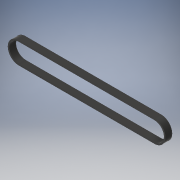
# Autodesk Inventor part: BeltVer1-1111-2019
Saved by Autodesk Inventor 2018 (Build 220112000, 112)
## iProperties
Created: 2018-01-17
Part Number: BeltVer1-1111-2019
Material: Fiberglass Batt
Document SubType Name: Modeling
Designer: Sean
Density: 0.032 g/cm^3
Appearance: Smooth - Black
Mass: 1.04183 g
Surface Area: 280.777 cm^2
Volume: 32.5573 cm^3
Author: Sean
Autodesk Inventor part; units mm, degrees
ref_plane "YZ Plane" through (0, 0, 0) normal (1, 0, 0) x (0, 1, 0)
ref_plane "XZ Plane" through (0, 0, 0) normal (0, 1, 0) x (-1, 0, 0)
ref_plane "XY Plane" through (0, 0, 0) normal (0, 0, 1) x (1, 0, 0)
sketch "Sketch1" plane through (0, 0, 0) normal (0, 0, 1) x (1, 0, 0)
  line L0 (0, 0) -> (301.6504, 0) construction
  line L1 (0, -23.2918) -> (301.6504, -23.2918)
  line L2 (301.6504, 23.2918) -> (0, 23.2918)
  arc A0 (0, 23.2918) -> (0, -23.2918) centre (0, 0) ccw
  arc A1 (301.6504, -23.2918) -> (301.6504, 23.2918) centre (301.6504, 0) ccw
  line L3 (0, 24.2062) -> (301.6504, 24.2062)
  arc A2 (301.6504, -24.2062) -> (301.6504, 24.2062) centre (301.6504, 0) ccw
  line L4 (301.6504, -24.2062) -> (0, -24.2062)
  arc A3 (0, 24.2062) -> (0, -24.2062) centre (0, 0) ccw
  line L5 (0, 21.463) -> (301.6504, 21.463)
  arc A4 (301.6504, -21.463) -> (301.6504, 21.463) centre (301.6504, 0) ccw
  line L6 (301.6504, -21.463) -> (0, -21.463)
  arc A5 (0, 21.463) -> (0, -21.463) centre (0, 0) ccw
  point P0 (150.8252, 0)
  dimension "d0" = 301.6504
  dimension "d1" = 23.2918
  dimension "d2" = 0.9144
  dimension "d3" = 1.8288
  constraints: 16 end point, 12 point on circle, 6 centre point, 4 tangent, 3 parallel, 1 horizontal, 1 midpoint, 6 other
  measures "d0" distance of L0.start L0.end
  measures "d1" distance between parallel lines of L2 L0
  measures "d2" distance between parallel lines of L3 L2
  measures "d3" distance between parallel lines of L2 L5
extrude "Extrusion1" add sketch "Sketch1" along normal blind 15 contours A0 L2 A1 L1 | L3 A2 L4 A3
body "Solid1"
